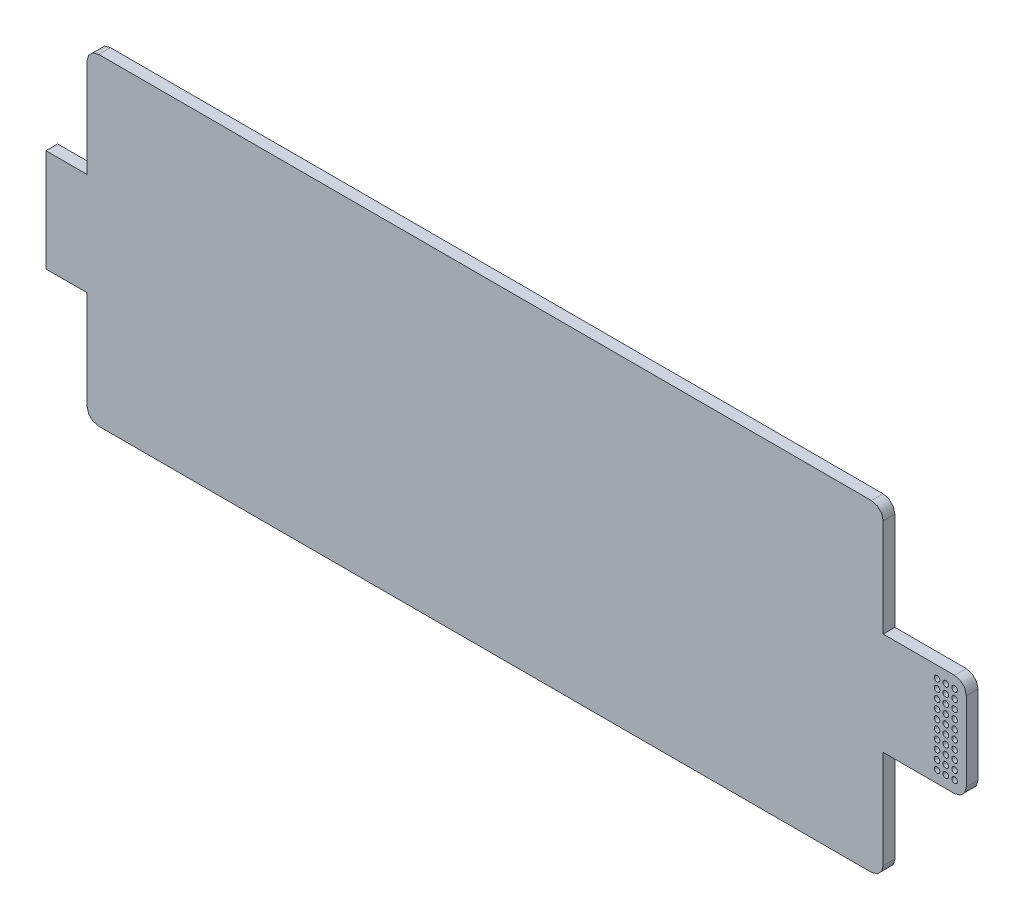
# Autodesk Inventor part: LogicPCB
Saved by Autodesk Inventor 2016 (Build 200138000, 138)
## iProperties
Created: 2015-06-09
Part Number: LogicPCB
Material: GFRC
Document SubType Name: Modeling
Designer: Yann
Density: 1.7 g/cm^3
Appearance: Flat - Polished Gray
Author: Yann
Autodesk Inventor part; units mm, degrees
ref_plane "YZ Plane" through (0, 0, 0) normal (1, 0, 0) x (0, 1, 0)
ref_plane "XZ Plane" through (0, 0, 0) normal (0, 1, 0) x (-1, 0, 0)
ref_plane "XY Plane" through (0, 0, 0) normal (0, 0, 1) x (1, 0, 0)
sketch "Sketch1" plane through (0, 0, 0) normal (0, 0, 1) x (1, 0, 0)
  line L0 (0, 39.0799) -> (0, -39.0799) construction
  line L1 (-106.5228, 0) -> (114.1371, 0) construction
  line L2 (0, 27.5) -> (66, 27.5)
  line L3 (68, 25.5) -> (68, 8.75)
  line L4 (68, 8.75) -> (80.2, 8.75)
  line L5 (82.2, 6.75) -> (82.2, 0)
  line L6 (75, 22.5739) -> (75, -22.5739) construction
  circle A0 centre (77.2, 6.75) radius 0.5
  circle A1 centre (78.7, 6.75) radius 0.5
  circle A2 centre (80.2, 6.75) radius 0.5
  circle A3 centre (77.2, 5.25) radius 0.5
  circle A4 centre (78.7, 5.25) radius 0.5
  circle A5 centre (80.2, 5.25) radius 0.5
  circle A6 centre (77.2, 3.75) radius 0.5
  circle A7 centre (78.7, 3.75) radius 0.5
  circle A8 centre (80.2, 3.75) radius 0.5
  circle A9 centre (77.2, 2.25) radius 0.5
  circle A10 centre (78.7, 2.25) radius 0.5
  circle A11 centre (80.2, 2.25) radius 0.5
  circle A12 centre (77.2, 0.75) radius 0.5
  circle A13 centre (78.7, 0.75) radius 0.5
  circle A14 centre (80.2, 0.75) radius 0.5
  circle A15 centre (77.2, -0.75) radius 0.5
  circle A16 centre (78.7, -0.75) radius 0.5
  circle A17 centre (80.2, -0.75) radius 0.5
  circle A18 centre (77.2, -2.25) radius 0.5
  circle A19 centre (78.7, -2.25) radius 0.5
  circle A20 centre (80.2, -2.25) radius 0.5
  circle A21 centre (77.2, -3.75) radius 0.5
  circle A22 centre (78.7, -3.75) radius 0.5
  circle A23 centre (80.2, -3.75) radius 0.5
  circle A24 centre (77.2, -5.25) radius 0.5
  circle A25 centre (78.7, -5.25) radius 0.5
  circle A26 centre (80.2, -5.25) radius 0.5
  circle A27 centre (77.2, -6.75) radius 0.5
  circle A28 centre (78.7, -6.75) radius 0.5
  circle A29 centre (80.2, -6.75) radius 0.5
  arc A30 (82.2, 6.75) -> (80.2, 8.75) centre (80.2, 6.75) ccw
  arc A31 (68, 25.5) -> (66, 27.5) centre (66, 25.5) ccw
  line L7 (0, -27.5) -> (66, -27.5)
  line L8 (68, -25.5) -> (68, -8.75)
  line L9 (68, -8.75) -> (80.2, -8.75)
  line L10 (82.2, -6.75) -> (82.2, 0)
  line L11 (75, -22.5739) -> (75, 22.5739) construction
  arc A32 (80.2, -8.75) -> (82.2, -6.75) centre (80.2, -6.75) ccw
  arc A33 (66, -27.5) -> (68, -25.5) centre (66, -25.5) ccw
  line L12 (0, 27.5) -> (-66, 27.5)
  line L13 (-68, 25.5) -> (-68, 8.75)
  arc A34 (-66, 27.5) -> (-68, 25.5) centre (-66, 25.5) ccw
  line L14 (0, -27.5) -> (-66, -27.5)
  line L15 (-68, -25.5) -> (-68, -8.75)
  arc A35 (-68, -25.5) -> (-66, -27.5) centre (-66, -25.5) ccw
  line L16 (-75, -22.5739) -> (-75, 22.5739) construction
  line L17 (-68, 8.75) -> (-75, 8.75)
  line L18 (-75, 8.75) -> (-75, -8.75)
  line L19 (-68, -8.75) -> (-75, -8.75)
  point P0 (0, 0)
  dimension "d0" = 27.5
  dimension "d1" = 7
  dimension "d2" = 1
  dimension "d5" = 1.5
  dimension "d8" = 1.5
  dimension "d11" = 2
  dimension "d12" = 2
  dimension "d13" = 2
  dimension "d15" = 2.2
  dimension "d16" = 2
  constraints: 36 centre point, 30 end point, 19 symmetric about line, 12 point on circle, 5 perpendicular, 4 point on line, 4 tangent, 2 horizontal, 1 vertical, 62 other
  measures "d0" distance between parallel lines of L1 L2
  measures "d1" distance between parallel lines of L3 L6
  measures "d2" diameter of A0
  measures "d5" distance of A0.centre A1.centre
  measures "d8" distance of A0.centre A3.centre
  measures "d11" distance from line of L5 A17.centre
  measures "d12" distance from line of L4 A2.centre
  measures "d13" radius of A30
  measures "d15" distance from line of L6 A3.centre
  measures "d16" radius of A31
extrude "Extrusion1" add sketch "Sketch1" along normal blind 2
equation "\"d0\" = 0.5 * LogicPCB_Width"
equation "\"d1\" = Interface_Thickness"
equation "\"d12\" = d11"
equation "\"d17\" = LogicPCB_Thickness"
equation "\"Heatsink_Thickness\" = 5"
equation "\"Heatsink_Width\" = 65"
equation "\"Cover_Thickness\" = 2"
equation "\"PowerPCB_Minus_Height\" = 1.2"
equation "\"PowerPCB_Width\" = 63"
equation "\"Interface_Thickness\" = 7"
equation "\"PowerPCB_Thickness\" = 3"
equation "\"PowerPCB_Plus_Height\" = 8"
equation "\"LogicPCB_Width\" = 55"
equation "\"LogicPCB_Thickness\" = 2"
equation "\"LogicPCB_Plus_Height\" = 8"
equation "\"HostPCB_Plus_Height\" = 8"
equation "\"HostPCB_Thickness\" = 1.2"
body "Solid1"
